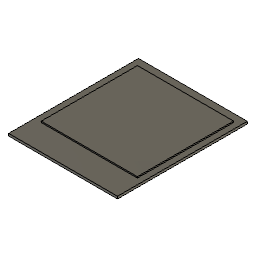
Watch (Autodesk Fusion 360 archive; units mm, degrees)
design "Display"
part number: 2026-04-19-13-29-12-913
Autodesk Fusion 360 part; units mm, degrees
sketch "Sketch1" plane through (0, 0, 0) normal (0, 0, 1) x (1, 0, 0)
  line L0 (0, 0) -> (31.2788, 0)
  line L1 (31.2788, 0) -> (31.2788, 37.3)
  line L2 (31.2788, 37.3) -> (0, 37.3)
  line L3 (0, 37.3) -> (0, 0)
  dimension "d1" = 37.3
  constraint horizontal L0
  constraint vertical L1
  constraint horizontal L2
  constraint vertical L3
  constraint coincident L0.start L3.end
  measures "d1" distance of L0.start L2.end
extrude "Extrude1" add sketch "Sketch1" along normal blind 0.7
sketch "Sketch2" plane through (0, 0, 0.7) normal (0, 0, 1) x (-1, 0, 0)
  line L0 (0, -37.3) -> (0, 0)
  line L1 (0, 0) -> (-31.2788, 0)
  line L2 (-31.2788, 0) -> (-31.2788, -37.3)
  line L3 (-31.2788, -37.3) -> (0, -37.3)
  line L4 (-2, -35) -> (-29.6, -35)
  line L5 (-29.6, -35) -> (-29.6, -7.3786)
  line L6 (-29.6, -7.3786) -> (-2, -7.3786)
  line L7 (-2, -7.3786) -> (-2, -35)
  dimension "d4" = 27.6
  constraint horizontal L4
  constraint vertical L5
  constraint horizontal L6
  constraint vertical L7
  measures "d4" distance of L4.start L4.end
extrude "Extrude2" add sketch "Sketch2" along normal blind 0.35 contours L4 L5 L6 L7

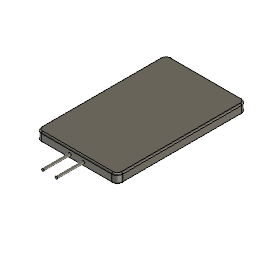
design "Battery"
part number: 2026-04-15-17-01-45-007
Autodesk Fusion 360 part; units mm, degrees
sketch "Sketch2" plane through (0, 0, 0) normal (0, 0, 1) x (1, 0, 0)
  line L0 (0, 0) -> (30.0402, 0)
  line L1 (30.0402, 0) -> (30.0402, 48)
  line L2 (30.0402, 48) -> (0, 48)
  line L3 (0, 48) -> (0, 0)
  dimension "d2" = 48
  constraint horizontal L0
  constraint vertical L1
  constraint horizontal L2
  constraint vertical L3
  constraint coincident L0.start L3.end
  measures "d2" distance of L0.start L2.end
extrude "Extrude1" add sketch "Sketch2" along normal blind 3.5
fillet "Fillet1" radius 2 4 edges at (0, 0, 1.75) (0, 48, 1.75) (30.0402, 48, 1.75) (30.0402, 0, 1.75)
fillet "Fillet2" radius 0.5 16 edges at (0.5858, 0.5858, 3.5) (15.0201, 0, 3.5) (29.4544, 0.5858, 3.5) (30.0402, 24, 3.5) (29.4544, 47.4142, 3.5) (15.0201, 48, 3.5) (0.5858, 47.4142, 3.5) (0, 24, 3.5) (15.0201, 0, 0) (29.4544, 0.5858, 0) (30.0402, 24, 0) (29.4544, 47.4142, 0) (15.0201, 48, 0) (0.5858, 47.4142, 0) (0, 24, 0) (0.5858, 0.5858, 0)
sketch "Sketch3" plane through (0, 0, 0) normal (0, -1, 0) x (1, 0, 0)
  line L0 (2, 0.5) -> (28.0402, 0.5)
  line L1 (28.0402, 0.5) -> (28.0402, 3)
  line L2 (28.0402, 3) -> (2, 3)
  line L3 (2, 3) -> (2, 0.5)
  circle A0 centre (12.5201, 1.5908) radius 0.5
  circle A1 centre (17.5201, 1.5908) radius 0.5
  line L4 (15.0201, 3) -> (15.0201, 0.5)
  dimension "d9" = 1
  dimension "d10" = 1
  dimension "d11" = 5
  constraint horizontal A0.centre A1.centre
  constraint midpoint L2 L4.start
  constraint midpoint L0 L4.end
  constraint symmetric A0.centre A1.centre L4
  measures "d9" diameter of A0
  measures "d10" diameter of A1
  measures "d11" distance of A0.centre A1.centre
extrude "Extrude2" add sketch "Sketch3" along normal blind 10 contours A0 | A1
